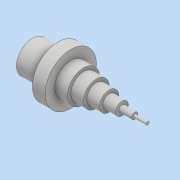
# Autodesk Inventor part: P3
Saved by Autodesk Inventor 2017 (Build 210142000, 142)
## iProperties
Part Number: P3
Material: 一般
Document SubType Name: Modeling
Designer: d8910
Density: 1 g/cm^3
Appearance: 預設
Author: d8910
Autodesk Inventor part; units mm, degrees
ref_plane "YZ Plane" through (0, 0, 0) normal (1, 0, 0) x (0, 1, 0)
ref_plane "XZ Plane" through (0, 0, 0) normal (0, 1, 0) x (-1, 0, 0)
ref_plane "XY Plane" through (0, 0, 0) normal (0, 0, 1) x (1, 0, 0)
sketch "草圖1" plane through (0, 0, 0) normal (0, 0, 1) x (1, 0, 0)
  line L0 (-80, 0) -> (-40, 0)
  line L1 (-40, 0) -> (-40, 25)
  line L2 (-40, 25) -> (-80, 25)
  line L3 (-80, 25) -> (-80, 0)
  line L4 (-40, 0) -> (-20, 0)
  line L5 (-20, 0) -> (-20, 40)
  line L6 (-20, 40) -> (-40, 40)
  line L7 (-40, 40) -> (-40, 0)
  line L8 (-20, 0) -> (0, 0)
  line L9 (0, 0) -> (0, 25)
  line L10 (0, 25) -> (-20, 25)
  line L11 (-20, 25) -> (-20, 0)
  line L12 (0, 0) -> (20, 0)
  line L13 (20, 0) -> (20, 20)
  line L14 (20, 20) -> (0, 20)
  line L15 (0, 20) -> (0, 0)
  line L16 (20, 0) -> (40, 0)
  line L17 (40, 0) -> (40, 15)
  line L18 (40, 15) -> (20, 15)
  line L19 (20, 15) -> (20, 0)
  line L20 (40, 0) -> (60, 0)
  line L21 (60, 0) -> (60, 10)
  line L22 (60, 10) -> (40, 10)
  line L23 (40, 10) -> (40, 0)
  line L24 (60, 0) -> (80, 0)
  line L25 (80, 0) -> (80, 5)
  line L26 (80, 5) -> (60, 5)
  line L27 (60, 5) -> (60, 0)
  line L28 (80, 0) -> (100, 0)
  line L29 (100, 0) -> (100, 2.5)
  line L30 (100, 2.5) -> (80, 2.5)
  line L31 (80, 2.5) -> (80, 0)
  line L32 (-80, 0) -> (-40, 0)
  line L33 (-40, 0) -> (-40, 20)
  line L34 (-40, 20) -> (-80, 20)
  line L35 (-80, 20) -> (-80, 0)
  line L36 (-40, 40) -> (-20, 40)
  line L37 (-20, 40) -> (-20, 0)
  line L38 (-20, 0) -> (-40, 0)
  line L39 (-40, 0) -> (-40, 40)
  dimension "d0" = 20
  dimension "d1" = 25
  dimension "d2" = 40
  dimension "d3" = 25
  dimension "d4" = 20
  dimension "d5" = 15
  dimension "d6" = 10
  dimension "d7" = 5
  dimension "d8" = 2.5
  dimension "d9" = 40
  dimension "d10" = 180
  dimension "d11" = 20
  dimension "d12" = 20
  dimension "d13" = 20
  dimension "d14" = 20
  dimension "d15" = 20
  dimension "d16" = 20
  constraints: 80 end point, 20 parallel, 10 horizontal, 10 perpendicular, 2 horizontal alignment, 1 midpoint, 1 vertical alignment
  measures "d0" distance between parallel lines of L0 L34
  measures "d1" distance between parallel lines of L2 L0
  measures "d2" distance between parallel lines of L4 L6
  measures "d3" distance between parallel lines of L10 L8
  measures "d4" distance between parallel lines of L12 L14
  measures "d5" distance between parallel lines of L16 L18
  measures "d6" distance between parallel lines of L20 L22
  measures "d7" distance between parallel lines of L24 L26
  measures "d8" distance between parallel lines of L28 L30
  measures "d9" distance of L1.end L2.end
  measures "d10" distance between parallel lines of L3 L29
  measures "d11" distance of L29.end L30.end
  measures "d12" distance of L25.end L26.end
  measures "d13" distance of L21.end L22.end
  measures "d14" distance of L17.end L18.end
  measures "d15" distance of L13.end L14.end
  measures "d16" distance of L9.end L10.end
revolve "迴轉1" add sketch "草圖1" angle 360 about axis through (-80, 0, 0) along (1, 0, 0) contours L1 L7 L6 L5 L4 | L3 L2 L1 L34 | L5 L10 L9 L8 | L9 L14 L13 L12 | L13 L18 L17 L16 | L17 L22 L21 L20 | L21 L26 L25 L24 | L25 L30 L29 L28
